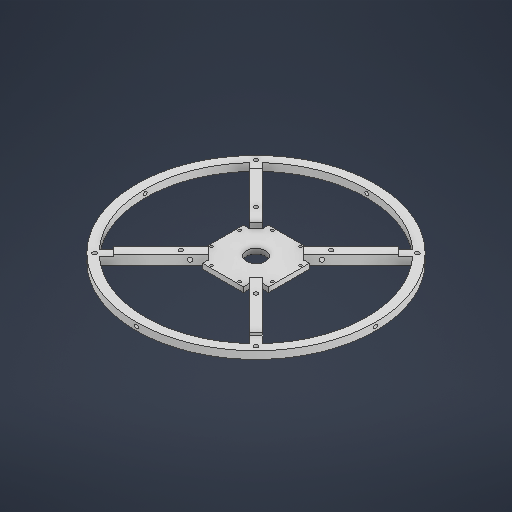
# Autodesk Inventor part: podstawa-serwomechanizmy
Saved by Autodesk Inventor 2026.2 (Build 302298010, 298A)
## iProperties
Created: 2026-04-18
Part Number: podstawa-serwomechanizmy
Material: Ogólny
Document SubType Name: Modeling
Designer: macie
Density: 1 g/cm^3
Appearance: Domyślna
Author: macie
Autodesk Inventor part; units mm, degrees
ref_plane "YZ Plane" through (0, 0, 0) normal (1, 0, 0) x (0, 1, 0)
ref_plane "XZ Plane" through (0, 0, 0) normal (0, 1, 0) x (-1, 0, 0)
ref_plane "XY Plane" through (0, 0, 0) normal (0, 0, 1) x (1, 0, 0)
sketch "Szkic1" plane through (0, 0, 0) normal (0, 1, 0) x (-1, 0, 0)
  circle A0 centre (0, 0) radius 27
  circle A1 centre (0, 0) radius 7.5
  dimension "d0" = 54
  dimension "d1" = 15
  constraints: 2 centre point, 2 coincident
  measures "d0" diameter of A0
  measures "d1" diameter of A1
extrude "Wyciągnięcie proste1" add sketch "Szkic1" along normal blind 4
sketch "Szkic2" plane through (0, 4, 0) normal (0, 1, 0) x (1, 0, 0)
  circle A0 centre (0, 0) radius 27 projected
  line L0 (26.2667, -6.25) -> (26.2667, 6.25)
  line L1 (26.2667, 6.25) -> (21.2667, 6.25)
  line L2 (21.2667, 6.25) -> (21.2667, -6.25)
  line L3 (21.2667, -6.25) -> (26.2667, -6.25)
  line L4 (6.25, 26.2667) -> (-6.25, 26.2667)
  line L5 (-6.25, 21.2667) -> (6.25, 21.2667)
  line L6 (6.25, 21.2667) -> (6.25, 26.2667)
  line L7 (-6.25, 26.2667) -> (-6.25, 21.2667)
  line L8 (-26.2667, 6.25) -> (-26.2667, -6.25)
  line L9 (-21.2667, -6.25) -> (-21.2667, 6.25)
  line L10 (-21.2667, 6.25) -> (-26.2667, 6.25)
  line L11 (-26.2667, -6.25) -> (-21.2667, -6.25)
  line L12 (-6.25, -26.2667) -> (6.25, -26.2667)
  line L13 (6.25, -21.2667) -> (-6.25, -21.2667)
  line L14 (-6.25, -21.2667) -> (-6.25, -26.2667)
  line L15 (6.25, -26.2667) -> (6.25, -21.2667)
  point P0 (-6.25, 26.2667)
  point P1 (6.25, 26.2667)
  point P2 (-26.2667, -6.25)
  point P3 (-26.2667, 6.25)
  point P4 (6.25, -26.2667)
  point P5 (-6.25, -26.2667)
  dimension "d4" = 5
  dimension "d5" = 12.5
  dimension "d8" = 360
  constraints: 32 end point, 2 parallel, 2 point on circle, 1 perpendicular, 1 vertical, 33 other
  measures "d4" distance between parallel lines of L2 L0
  measures "d5" distance between parallel lines of L1 L3
extrude "Wyciągnięcie proste2" cut sketch "Szkic2" against normal blind 4 contours A0 L0 | L4 A0 | A0 L12 | L8 A0
sketch "Szkic3" plane through (0, 4, 0) normal (0, 1, 0) x (1, 0, 0)
  line L0 (26.2667, 6.25) -> (26.2667, -6.25) projected
  line L1 (26.2667, 6.25) -> (21.2667, 6.25)
  line L2 (21.2667, 6.25) -> (21.2667, -6.25)
  line L3 (21.2667, -6.25) -> (26.2667, -6.25)
  line L4 (26.2667, -6.25) -> (26.2667, 6.25)
  line L5 (21.2667, -6.25) -> (25.2667, -6.25)
  line L6 (25.2667, -6.25) -> (25.2667, -9.25)
  line L7 (25.2667, -9.25) -> (21.2667, -9.25)
  line L8 (21.2667, -9.25) -> (21.2667, -6.25)
  line L9 (26.2667, -6.25) -> (6.4667, -6.25)
  line L10 (6.4667, -6.25) -> (6.4667, 6.25)
  line L11 (6.4667, 6.25) -> (26.2667, 6.25)
  line L12 (26.2667, 6.25) -> (26.2667, -6.25)
  circle A0 centre (0, 0) radius 7.5 projected
  line L13 (26.2667, -6.25) -> (24.2667, -6.25)
  line L14 (24.2667, -6.25) -> (24.2667, -11.25)
  line L15 (24.2667, -11.25) -> (26.2667, -11.25)
  line L16 (26.2667, -11.25) -> (26.2667, -6.25)
  line L17 (26.2667, -6.25) -> (21.2667, -6.25)
  line L18 (21.2667, -6.25) -> (21.2667, -16.25)
  line L19 (21.2667, -16.25) -> (26.2667, -16.25)
  line L20 (26.2667, -16.25) -> (26.2667, -6.25)
  line L21 (0, 0) -> (26.2667, 0)
  line L22 (25.2667, 6.25) -> (25.2667, 9.25)
  line L23 (25.2667, 9.25) -> (21.2667, 9.25)
  line L24 (24.2667, 6.25) -> (24.2667, 11.25)
  line L25 (24.2667, 11.25) -> (26.2667, 11.25)
  line L26 (21.2667, 6.25) -> (21.2667, 16.25)
  line L27 (21.2667, 16.25) -> (26.2667, 16.25)
  line L28 (26.2667, 16.25) -> (26.2667, 6.25)
  line L29 (-6.25, 26.2667) -> (-6.25, 21.2667)
  line L30 (-9.25, 25.2667) -> (-9.25, 21.2667)
  line L31 (-6.25, 25.2667) -> (-9.25, 25.2667)
  line L32 (-11.25, 24.2667) -> (-11.25, 26.2667)
  line L33 (-6.25, 24.2667) -> (-11.25, 24.2667)
  line L34 (-6.25, 21.2667) -> (-16.25, 21.2667)
  line L35 (-16.25, 21.2667) -> (-16.25, 26.2667)
  line L36 (-16.25, 26.2667) -> (-6.25, 26.2667)
  line L37 (6.25, 21.2667) -> (6.25, 26.2667)
  line L38 (6.25, 25.2667) -> (9.25, 25.2667)
  line L39 (9.25, 25.2667) -> (9.25, 21.2667)
  line L40 (9.25, 21.2667) -> (6.25, 21.2667)
  line L41 (6.25, 24.2667) -> (11.25, 24.2667)
  line L42 (11.25, 24.2667) -> (11.25, 26.2667)
  line L43 (11.25, 26.2667) -> (6.25, 26.2667)
  line L44 (6.25, 21.2667) -> (16.25, 21.2667)
  line L45 (16.25, 26.2667) -> (6.25, 26.2667)
  line L46 (16.25, 21.2667) -> (16.25, 26.2667)
  line L47 (6.25, 26.2667) -> (6.25, 24.2667)
  line L48 (6.25, 26.2667) -> (6.25, 21.2667)
  line L49 (6.25, 21.2667) -> (6.25, 25.2667)
  line L50 (-26.2667, -6.25) -> (-21.2667, -6.25)
  line L51 (-25.2667, -9.25) -> (-21.2667, -9.25)
  line L52 (-25.2667, -6.25) -> (-25.2667, -9.25)
  line L53 (-24.2667, -11.25) -> (-26.2667, -11.25)
  line L54 (-24.2667, -6.25) -> (-24.2667, -11.25)
  line L55 (-21.2667, -6.25) -> (-21.2667, -16.25)
  line L56 (-21.2667, -16.25) -> (-26.2667, -16.25)
  line L57 (-26.2667, -16.25) -> (-26.2667, -6.25)
  line L58 (-21.2667, 6.25) -> (-26.2667, 6.25)
  line L59 (-25.2667, 6.25) -> (-25.2667, 9.25)
  line L60 (-25.2667, 9.25) -> (-21.2667, 9.25)
  line L61 (-21.2667, 9.25) -> (-21.2667, 6.25)
  line L62 (-24.2667, 6.25) -> (-24.2667, 11.25)
  line L63 (-24.2667, 11.25) -> (-26.2667, 11.25)
  line L64 (-26.2667, 11.25) -> (-26.2667, 6.25)
  line L65 (-21.2667, 6.25) -> (-21.2667, 16.25)
  line L66 (-26.2667, 16.25) -> (-26.2667, 6.25)
  line L67 (-21.2667, 16.25) -> (-26.2667, 16.25)
  line L68 (-26.2667, 6.25) -> (-24.2667, 6.25)
  line L69 (-26.2667, 6.25) -> (-21.2667, 6.25)
  line L70 (-21.2667, 6.25) -> (-25.2667, 6.25)
  line L71 (6.25, -26.2667) -> (6.25, -21.2667)
  line L72 (9.25, -25.2667) -> (9.25, -21.2667)
  line L73 (6.25, -25.2667) -> (9.25, -25.2667)
  line L74 (11.25, -24.2667) -> (11.25, -26.2667)
  line L75 (6.25, -24.2667) -> (11.25, -24.2667)
  line L76 (6.25, -21.2667) -> (16.25, -21.2667)
  line L77 (16.25, -21.2667) -> (16.25, -26.2667)
  line L78 (16.25, -26.2667) -> (6.25, -26.2667)
  line L79 (-6.25, -21.2667) -> (-6.25, -26.2667)
  line L80 (-6.25, -25.2667) -> (-9.25, -25.2667)
  line L81 (-9.25, -25.2667) -> (-9.25, -21.2667)
  line L82 (-9.25, -21.2667) -> (-6.25, -21.2667)
  line L83 (-6.25, -24.2667) -> (-11.25, -24.2667)
  line L84 (-11.25, -24.2667) -> (-11.25, -26.2667)
  line L85 (-11.25, -26.2667) -> (-6.25, -26.2667)
  line L86 (-6.25, -21.2667) -> (-16.25, -21.2667)
  line L87 (-16.25, -26.2667) -> (-6.25, -26.2667)
  line L88 (-16.25, -21.2667) -> (-16.25, -26.2667)
  line L89 (-6.25, -26.2667) -> (-6.25, -24.2667)
  line L90 (-6.25, -26.2667) -> (-6.25, -21.2667)
  line L91 (-6.25, -21.2667) -> (-6.25, -25.2667)
  point P0 (23.2667, -9.25)
  point P1 (21.2667, -7.75)
  point P2 (25.2667, -7.75)
  point P3 (6.25, -26.2667)
  point P4 (-6.25, 26.2667)
  point P5 (7.75, 21.2667)
  point P6 (7.75, 25.2667)
  point P7 (9.25, 23.2667)
  point P8 (-26.2667, -6.25)
  point P9 (-21.2667, 7.75)
  point P10 (-25.2667, 7.75)
  point P11 (-23.2667, 9.25)
  point P12 (6.25, -26.2667)
  point P13 (-7.75, -21.2667)
  point P14 (-7.75, -25.2667)
  point P15 (-9.25, -23.2667)
  dimension "d12" = 5
  dimension "d13" = 12.5
  dimension "d14" = 3
  dimension "d15" = 4
  dimension "d18" = 19.8
  dimension "d22" = 12.5
  dimension "d23" = 2
  dimension "d24" = 5
  dimension "d25" = 5
  dimension "d26" = 5
  dimension "d29" = 360
  constraints: 182 end point, 10 parallel, 10 symmetric about line, 5 horizontal, 5 perpendicular, 4 midpoint, 193 other
  measures "d12" distance between parallel lines of L0 L2
  measures "d13" distance between parallel lines of L3 L1
  measures "d14" distance from line of point (23.267, -9.25) L3
  measures "d15" distance of point (21.267, -7.75) point (25.267, -7.75)
  measures "d18" distance between parallel lines of L0 L10
  measures "d22" distance between parallel lines of L9 L11
  measures "d23" distance of L15.end L14.end
  measures "d24" distance between parallel lines of L15 L5
  measures "d25" distance between parallel lines of L20 L18
  measures "d26" distance between parallel lines of L15 L19
extrude "Wyciągnięcie proste5" add sketch "Szkic3" against normal blind 4 contours L1 L22 L23 L24 L25 L28 | L25 L24 L23 L26 L27 L28 | L16 L15 L14 L7 L6 L3 | L20 L19 L18 L7 L14 L15 | L29 L31 L30 L33 L32 L36 | L32 L33 L30 L34 L35 L36 | L39 L41 L42 L45 L46 L44 | L37 L43 L42 L41 L39 L38 | L50 L52 L51 L54 L53 L57 | L53 L54 L51 L55 L56 L57 | L60 L62 L63 L66 L67 L65 | L58 L64 L63 L62 L60 L59 | L71 L73 L72 L75 L74 L78 | L74 L75 L72 L76 L77 L78 | L81 L83 L84 L87 L88 L86 | L79 L85 L84 L83 L81 L80
hole "Otwór1" at (24.2667, 4, 11.25) at (24.2667, 4, -11.25) at (-11.25, 4, -24.2667) at (11.25, 4, -24.2667) at (-24.2667, 4, 11.25) at (-24.2667, 4, -11.25) at (11.25, 4, 24.2667) at (-11.25, 4, 24.2667) direction (0, -1, 0) diameter 2.2 end through all
sketch "Szkic4" plane through (0, 4, 0) normal (0, 1, 0) x (1, 0, 0)
  line L0 (-21.5624, 16.25) -> (-26.2667, 16.25) projected
  line L1 (-21.5624, 16.25) -> (-59.2247, 53.9123)
  arc A0 (-16.25, 21.5624) -> (-21.5624, 16.25) centre (0, 0) ccw projected
  line L2 (-16.25, 21.5624) -> (-53.9123, 59.2247)
  line L3 (-59.2247, 53.9123) -> (-53.9123, 59.2247)
  line L4 (0, 0) -> (-73.6398, 0)
  line L5 (-21.5624, -16.25) -> (-59.2247, -53.9123)
  line L6 (-53.9123, -59.2247) -> (-59.2247, -53.9123)
  line L7 (-16.25, -21.5624) -> (-53.9123, -59.2247)
  line L8 (16.25, -21.5624) -> (53.9123, -59.2247)
  line L9 (59.2247, -53.9123) -> (53.9123, -59.2247)
  line L10 (21.5624, -16.25) -> (59.2247, -53.9123)
  line L11 (21.5624, 16.25) -> (59.2247, 53.9123)
  line L12 (53.9123, 59.2247) -> (59.2247, 53.9123)
  line L13 (16.25, 21.5624) -> (53.9123, 59.2247)
  circle A1 centre (0, 0) radius 27
  dimension "d42" = 45
  dimension "d43" = 80
  dimension "d44" = 45
  dimension "d45" = 73.6398
  dimension "d48" = 360
  constraints: 26 end point, 1 coincident, 1 horizontal, 1 perpendicular, 32 other
  measures "d42" angle of L4 L1
  measures "d43" distance from line of L3 point (0, 0)
  measures "d44" angle of L2 L4
  measures "d45" distance of point (0, 0) L4.end
extrude "Wyciągnięcie proste6" add sketch "Szkic4" along normal blind 4 and the other way blind 4 contours L1 L3 L2 A0 | L13 L12 L11 A1 | A1 L7 L6 L5 | A1 L10 L9 L8
sketch "Szkic7" plane through (0, 4, 0) normal (0, 1, 0) x (1, 0, 0)
  line L0 (-53.9123, 59.2247) -> (-59.2247, 53.9123) projected
  line L1 (-59.2247, 53.9123) -> (-53.9123, 59.2247)
  line L2 (-53.9123, 59.2247) -> (-64.5189, 69.8313)
  line L3 (-64.5189, 69.8313) -> (-69.8313, 64.5189)
  line L4 (-69.8313, 64.5189) -> (-59.2247, 53.9123)
  line L5 (-59.2247, -53.9123) -> (-69.8313, -64.5189)
  line L6 (-64.5189, -69.8313) -> (-53.9123, -59.2247)
  line L7 (-53.9123, -59.2247) -> (-59.2247, -53.9123)
  line L8 (-69.8313, -64.5189) -> (-64.5189, -69.8313)
  line L9 (53.9123, -59.2247) -> (64.5189, -69.8313)
  line L10 (69.8313, -64.5189) -> (59.2247, -53.9123)
  line L11 (59.2247, -53.9123) -> (53.9123, -59.2247)
  line L12 (64.5189, -69.8313) -> (69.8313, -64.5189)
  line L13 (59.2247, 53.9123) -> (69.8313, 64.5189)
  line L14 (64.5189, 69.8313) -> (53.9123, 59.2247)
  line L15 (53.9123, 59.2247) -> (59.2247, 53.9123)
  line L16 (69.8313, 64.5189) -> (64.5189, 69.8313)
  circle A0 centre (0, 0) radius 95.0742
  circle A1 centre (0, 0) radius 7.5 projected
  circle A2 centre (0, 0) radius 88.0742
  point P0 (64.8774, 59.565)
  point P1 (64.8774, -59.565)
  point P2 (59.565, -64.8774)
  point P3 (-59.565, -64.8774)
  point P4 (-64.8774, -59.565)
  point P5 (-64.8774, 59.565)
  point P6 (-59.565, 64.8774)
  point P7 (59.565, 64.8774)
  dimension "d59" = 15
  dimension "d62" = 360
  dimension "d65" = 7
  constraints: 32 end point, 3 equal length, 2 coincident, 1 centre point, 1 perpendicular, 36 other
  measures "d59" distance between parallel lines of L0 L3
extrude "Wyciągnięcie proste7" add sketch "Szkic7" along normal blind 2 and the other way blind 4 contours L0 L4 A2 L2 | A2 L4 L3 L2 | L2 A0 L14 A2 | A2 L5 A0 L4 | L3 A0 | A2 L13 L15 L14 | L14 L16 L13 A2 | A2 L6 L8 L5 | L5 L7 L6 A2 | A0 L16 | L13 A0 L10 A2 | L8 A0 | A2 L9 A0 L6 | A2 L10 L12 L9 | L9 L11 L10 A2 | L12 A0
sketch "Szkic8" plane through (0, 6, 0) normal (0, 1, 0) x (1, 0, 0)
  line L0 (-21.5624, 16.25) -> (-64.8774, 59.565) projected
  line L1 (-59.565, 64.8774) -> (-16.25, 21.5624) projected
  line L2 (-64.8774, 59.565) -> (-59.565, 64.8774)
  line L3 (-59.565, 64.8774) -> (-64.5189, 69.8313)
  circle A0 centre (0, 0) radius 95.0742 projected
  line L4 (-64.8774, 59.565) -> (-69.8313, 64.5189)
  line L5 (-64.5189, 69.8313) -> (-64.8774, 59.565)
  line L6 (-59.565, 64.8774) -> (-69.8313, 64.5189)
  line L7 (-64.6982, 64.6982) -> (-62.2212, 62.2212)
  line L8 (-64.8774, 59.565) -> (-63.4597, 63.4597)
  line L9 (-63.4597, 63.4597) -> (-59.565, 64.8774)
  line L10 (-64.8774, 59.565) -> (-64.1688, 64.1688)
  line L11 (-64.1688, 64.1688) -> (-59.565, 64.8774)
  point P0 (-64.1688, -64.1688)
  point P1 (64.1688, -64.1688)
  point P2 (64.1688, 64.1688)
  dimension "d70" = 90
  dimension "d82" = 53.75
  dimension "d85" = 360
  constraints: 20 end point, 3 midpoint, 2 perpendicular, 2 point on circle, 1 coincident, 1 point on line, 5 other
  measures "d70" angle of L4 L2
  measures "d82" angle of L4 L10
hole "Otwór3" at (-64.1688, 6, -64.1688) at (64.1688, 6, -64.1688) at (64.1688, 6, 64.1688) at (-64.1688, 6, 64.1688) direction (0, -1, 0) diameter 3.2 end through all
sketch "Szkic13" plane through (16.25, 0, -21.5624) normal (-0.7071068, 0, -0.7071068) x (-0.7071068, 0, 0.7071068)
  line L0 (-3.3264, 4) -> (-3.3264, 0) projected
  line L1 (-53.2626, 8) -> (0, 8) projected
  line L2 (-3.3264, 0) -> (-3.3264, 8)
  line L3 (-3.3264, 8) -> (-10.3266, 8)
  line L4 (-10.3266, 8) -> (-10.3266, 0)
  line L5 (-10.3266, 0) -> (-3.3264, 0)
  point P0 (26.7374, 0)
  point P1 (-10.3266, 4)
  dimension "d123" = 37.064
  constraints: 8 end point, 2 parallel, 1 midpoint, 1 perpendicular, 1 point on line, 1 vertical
  measures "d123" distance from line of L4 point (26.737, 0)
hole "Otwór6" at (23.552, 4, -28.8644) direction (0.7071068, 0, 0.7071068) diameter 3.2 depth 8 tip angle 118
pattern_circular "Szyk kołowy1" count 4 over 360 about axis through (0, 0, 0) along (0, 1, 0) of "Otwór6"
sketch "Szkic15" plane through (0, 8, 0) normal (0, 1, 0) x (1, 0, 0)
  line L0 (-53.9123, -59.2247) -> (-16.25, -21.5624) projected
  point P0 (0, 0)
  point P1 (-29.8753, -29.8752)
  dimension "d134" = 42.25
  dimension "d135" = 3.7565
  measures "d134" distance of point (0, 0) point (-29.875, -29.875)
  measures "d135" distance from line of L0 point (-29.875, -29.875)
hole "Otwór7" at (-29.8753, 8, 29.8752) direction (0, -1, 0) diameter 3.2 end through all
pattern_circular "Szyk kołowy2" count 4 over 360 about axis through (0, 0, 0) along (0, 1, 0) of "Otwór7"
ref_plane "Płaszczyzna konstrukcyjna1" through (0, 4, 95.0742) normal (0, 0, 1) x (1, 0, 0)
sketch "Szkic16" plane through (0, 4, 95.0742) normal (0, 0, 1) x (1, 0, 0)
  line L0 (-95.0742, -4) -> (95.0742, -4) projected
  line L1 (-16.25, 0) -> (-16.25, 4) projected
  point P0 (0, -4)
  point P1 (0, -1)
  dimension "d146" = 3
  dimension "d147" = 16.25
  measures "d146" distance from line of L0 point (0, -1)
  measures "d147" distance from line of L1 point (0, -1)
hole "Otwór8" at (0, 3, 95.0742) direction (0, 0, -1) diameter 3 depth 8 tip angle 118
pattern_circular "Szyk kołowy3" count 4 over 360 about axis through (0, 0, 0) along (0, 1, 0) of "Otwór8"
equation "\"d22\" = d13"
equation "\"d26\" = d24"
